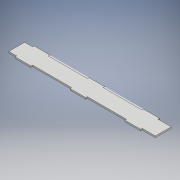
# Autodesk Inventor part: F5
Saved by Autodesk Inventor 2018 (Build 220112000, 112)
## iProperties
Created: 2018-03-06
Part Number: F5
Material: Generic
Document SubType Name: Modeling
Designer: isai
Density: 1 g/cm^3
Appearance: Default
Author: isai
Autodesk Inventor part; units mm, degrees
ref_plane "YZ Plane" through (0, 0, 0) normal (1, 0, 0) x (0, 1, 0)
ref_plane "XZ Plane" through (0, 0, 0) normal (0, 1, 0) x (-1, 0, 0)
ref_plane "XY Plane" through (0, 0, 0) normal (0, 0, 1) x (1, 0, 0)
sketch "Sketch1" plane through (0, 0, 0) normal (0, 0, 1) x (1, 0, 0)
  line L0 (-469, -128.2) -> (-449, -128.2)
  line L1 (-449, -128.2) -> (-449, -124.2)
  line L2 (-449, -124.2) -> (-409, -124.2)
  line L3 (-409, -124.2) -> (-409, -128.2)
  line L4 (-409, -128.2) -> (-309.6667, -128.2)
  line L5 (-309.6667, -128.2) -> (-309.6667, -124.2)
  line L6 (-309.6667, -124.2) -> (-269.6667, -124.2)
  line L7 (-269.6667, -124.2) -> (-269.6667, -128.2)
  line L8 (-269.6667, -128.2) -> (-170.3333, -128.2)
  line L9 (-170.3333, -128.2) -> (-170.3333, -124.2)
  line L10 (-170.3333, -124.2) -> (-130.3333, -124.2)
  line L11 (-130.3333, -124.2) -> (-130.3333, -128.2)
  line L12 (-130.3333, -128.2) -> (-101, -128.2)
  line L13 (-101, -128.2) -> (-97, -128.2)
  line L14 (-97, -128.2) -> (-97, -168.2)
  line L15 (-469, -128.2) -> (-469, -168.2)
  line L16 (-469, -148.2) -> (-507.0524, -148.2)
  line L17 (-269.6667, -172.2) -> (-269.6667, -168.2)
  line L18 (-130.3333, -172.2) -> (-130.3333, -168.2)
  line L19 (-170.3333, -168.2) -> (-170.3333, -172.2)
  line L20 (-170.3333, -172.2) -> (-130.3333, -172.2)
  line L21 (-449, -168.2) -> (-449, -172.2)
  line L22 (-449, -172.2) -> (-409, -172.2)
  line L23 (-309.6667, -172.2) -> (-269.6667, -172.2)
  line L24 (-309.6667, -168.2) -> (-309.6667, -172.2)
  line L25 (-409, -172.2) -> (-409, -168.2)
  line L26 (-449, -168.2) -> (-469, -168.2)
  line L27 (-309.6667, -168.2) -> (-409, -168.2)
  line L28 (-97, -168.2) -> (-130.3333, -168.2)
  line L29 (-170.3333, -168.2) -> (-269.6667, -168.2)
  point P0 (0, 0)
  dimension "d1" = 40
  constraints: 60 end point, 12 symmetric about line, 5 perpendicular, 2 horizontal, 1 midpoint, 1 vertical
  measures "d1" distance of L13.end L14.end
extrude "Extrusion2" add sketch "Sketch1" along normal blind 4
body "Solid2"
